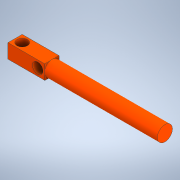
# Autodesk Inventor part: newblock
Saved by Autodesk Inventor 2022 (Build 260153000, 153)
## iProperties
Created: 2022-10-28
Part Number: newblock
Material: Generic
Document SubType Name: Modeling
Designer: matia
Density: 1 g/cm^3
Appearance: Default
Author: matia
Autodesk Inventor part; units mm, degrees
ref_plane "YZ Plane" through (0, 0, 0) normal (1, 0, 0) x (0, 1, 0)
ref_plane "XZ Plane" through (0, 0, 0) normal (0, 1, 0) x (-1, 0, 0)
ref_plane "XY Plane" through (0, 0, 0) normal (0, 0, 1) x (1, 0, 0)
sketch "Sketch1" plane through (0, 0, 0) normal (0, 1, 0) x (-1, 0, 0)
  line L0 (0, 0) -> (15.24, 0)
  circle A0 centre (15.24, 0) radius 3.556
  circle A1 centre (0, 0) radius 3.556
  line L1 (18.796, 0) -> (20.066, 0)
  line L2 (15.24, -3.556) -> (15.24, -4.826)
  line L3 (15.24, -4.826) -> (0, -4.826)
  line L4 (-3.556, 0) -> (-4.826, 0)
  line L5 (-4.826, 0) -> (-4.826, -4.826)
  line L6 (-4.826, -4.826) -> (0, -4.826)
  line L7 (15.24, -4.826) -> (20.066, -4.826)
  line L8 (20.066, -4.826) -> (20.066, 0)
  line L9 (15.24, 3.556) -> (15.24, 4.826)
  line L10 (15.24, 4.826) -> (20.066, 4.826)
  line L11 (20.066, 4.826) -> (-4.826, 4.826)
  line L12 (-4.826, 4.826) -> (-4.826, 0)
  line L13 (0, -4.826) -> (-4.826, -4.826)
  line L14 (20.066, 4.826) -> (20.066, 0)
  dimension "d2" = 7.112
  dimension "d0" = 15.24
  dimension "d1" = 7.112
  dimension "d3" = 1.27
  dimension "d4" = 1.27
  dimension "d5" = 1.27
  dimension "d6" = 1.27
  constraints: 30 end point, 7 perpendicular, 3 horizontal, 3 point on circle, 2 coincident, 2 point on line, 2 vertical, 1 centre point, 1 collinear, 1 horizontal alignment, 2 other
  measures "d0" distance of L0.start L0.end
  measures "d1" diameter of A0
  measures "d3" distance of L1.start L1.end
  measures "d4" distance of L2.start L2.end
  measures "d5" distance of L4.start L4.end
  measures "d6" distance of L9.start L9.end
extrude "Extrusion1" add sketch "Sketch1" along normal blind 9.652 contours A1 L4 L12 L11 L9 A0 L0 | A1 | L0 A0 L2 L3 L6 L5 L4 A1 | L9 L10 L14 L1 A0 | A0 L1 L8 L7 L2
sketch "Sketch2" plane through (4.826, 0, -4.826) normal (0, 0, -1) x (-1, 0, 0)
  line L0 (0, 0) -> (0, 9.652) projected
  line L1 (0, 4.826) -> (4.826, 4.826)
  circle A0 centre (4.826, 4.826) radius 3.556
  point P0 (4.826, 0)
  dimension "d9" = 4.826
  dimension "d10" = 7.112
  constraints: 2 end point, 1 centre point, 1 coincident, 1 horizontal, 1 midpoint
  measures "d9" distance of L1.start L1.end
  measures "d10" diameter of A0
extrude "Extrusion2" cut sketch "Sketch2" against normal through all
sketch "Sketch3" plane through (4.826, 0, 4.826) normal (1, 0, 0) x (0, 0, -1)
  line L0 (4.826, 0) -> (4.826, 9.652)
  line L1 (0, 9.652) -> (9.652, 9.652) projected
  line L2 (0, 0) -> (0, 9.652) projected
  line L3 (0, 4.826) -> (9.652, 4.826)
  line L4 (9.652, 0) -> (9.652, 9.652) projected
  circle A0 centre (4.826, 4.826) radius 5.08
  dimension "d13" = 10.16
  constraints: 4 end point, 4 midpoint, 1 centre point
  measures "d13" diameter of A0
extrude "Extrusion3" add sketch "Sketch3" along normal blind 76.2 contours L3 L2 A0 L1 L0 | L3 L4 A0 L2 | L0 L1 A0 L4 L3 | L1 A0 | L2 A0 | L4 A0
sketch "Sketch4" plane through (81.026, 4.826, 0) normal (1, 0, 0) x (0, 0, -1)
  circle A0 centre (0, 0) radius 5.08
  point P0 (0, -4.826)
  constraints: 1 centre point
extrude "Extrusion4" cut sketch "Sketch4" against normal blind 76.2
sketch "Sketch5" plane through (4.826, 0, 4.826) normal (1, 0, 0) x (0, 0, -1)
  line L0 (9.652, 9.652) -> (0, 9.652) projected
  line L1 (4.826, 9.652) -> (4.826, 0)
  circle A0 centre (4.826, 4.826) radius 5.08
  dimension "d18" = 10.16
  constraints: 2 end point, 2 midpoint, 1 centre point, 1 vertical
  measures "d18" diameter of A0
extrude "Extrusion5" add sketch "Sketch5" along normal blind 76.2
body "Solid1"
